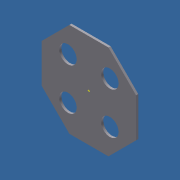
# Autodesk Inventor part: Stage2
Saved by Autodesk Inventor 2018.2 (Build 222227000, 227)
## iProperties
Created: 2018-10-31
Part Number: Stage2
Material: 3.3547 AlMg4,5Mn (AW-5083/H111)
Document SubType Name: Modeling
Designer: N.Grubert
Density: 2.66 g/cm^3
Appearance: Aluminum (gleichmäßig)
Fläche: 0 cm²
Gewicht: 0 g
Material: geeigneten Werkstoff auswählen !
Dateiname: P:\INVENTOR\Inventor 2018\Templates\ILT\Norm.ipt
Bez_eng: bolt
Bez_french: boulon
Author: N.Grubert
Autodesk Inventor part; units mm, degrees
ref_plane "YZ Plane" through (0, 0, 0) normal (1, 0, 0) x (0, 1, 0)
ref_plane "XZ Plane" through (0, 0, 0) normal (0, 1, 0) x (-1, 0, 0)
ref_plane "XY Plane" through (0, 0, 0) normal (0, 0, 1) x (1, 0, 0)
sketch "Skizze4" plane through (0, 0, 0) normal (0, 1, 0) x (-1, 0, 0)
  line L0 (-22.3675, 54) -> (22.3675, 54)
  line L1 (22.3675, 54) -> (54, 22.3675)
  line L2 (54, 22.3675) -> (54, -22.3675)
  line L3 (54, -22.3675) -> (22.3675, -54)
  line L4 (22.3675, -54) -> (-22.3675, -54)
  line L5 (-22.3675, -54) -> (-54, -22.3675)
  line L6 (-54, -22.3675) -> (-54, 22.3675)
  line L7 (-54, 22.3675) -> (-22.3675, 54)
  line L8 (75.6, 0) -> (-75.6, 0) construction
  line L9 (0, -75.6) -> (0, 75.6) construction
  circle A0 centre (-24, 24) radius 10
  circle A1 centre (-24, -24) radius 10
  circle A2 centre (24, -24) radius 10
  circle A3 centre (24, 24) radius 10
  point P0 (0, 0)
  point P1 (0, 0)
  dimension "d4" = 108
  dimension "d5" = 20
  dimension "d6" = 30
  dimension "d7" = 30
  dimension "d10" = 360
  constraints: 16 end point, 4 centre point, 1 coincident, 28 other
  measures "d4" distance between parallel lines of L4 L0
  measures "d5" diameter of A0
  measures "d6" distance from line of A0.centre L6
  measures "d7" distance from line of A0.centre L0
extrude "Extrusion2" add sketch "Skizze4" along normal blind 2.5
equation "\"d7\" = d6"
